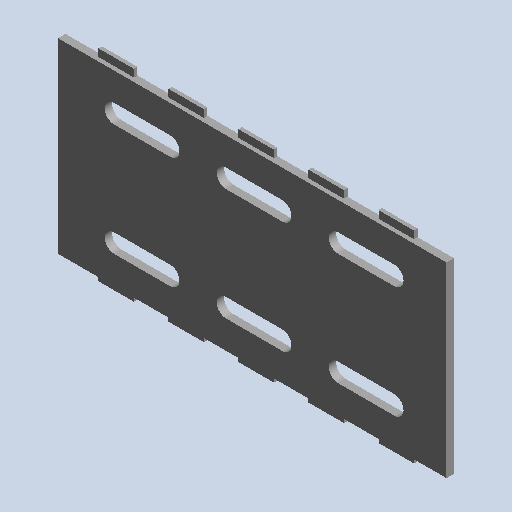
# Autodesk Inventor part: Enclosure_2
Saved by Autodesk Inventor 2026 (Build 300175050, 175E)
## iProperties
Part Number: Enclosure_2
Material: Generic
Document SubType Name: Modeling
Designer: Kartik
Mass: 75.559 g
Surface Area: 433.875 cm^2
Volume: 75.559 cm^3
Density: 1 g/cm^3
Appearance: Default
Author: Kartik
Autodesk Inventor part; units mm, degrees
ref_plane "YZ Plane" through (0, 0, 0) normal (1, 0, 0) x (0, 1, 0)
ref_plane "XZ Plane" through (0, 0, 0) normal (0, 1, 0) x (-1, 0, 0)
ref_plane "XY Plane" through (0, 0, 0) normal (0, 0, 1) x (1, 0, 0)
sketch "Sketch1" plane through (0, 0, 0) normal (0, 0, 1) x (1, 0, 0)
  line L0 (-100.0716, 53.5507) -> (107.9284, 53.5507)
  line L1 (107.9284, 53.5507) -> (107.9284, -46.4493)
  line L2 (107.9284, -46.4493) -> (-100.0716, -46.4493)
  line L3 (-100.0716, -46.4493) -> (-100.0716, 53.5507)
  point P0 (0, 0)
  dimension "d0" = 208
  dimension "d1" = 100
  constraints: 8 end point, 2 parallel, 1 horizontal, 1 perpendicular
  measures "d0" distance of L0.start L0.end
  measures "d1" distance of L0.end L1.end
extrude "Extrusion1" add sketch "Sketch1" along normal blind 4
sketch "Sketch2" plane through (-100.0716, -46.4493, 0) normal (0, -1, 0) x (1, 0, 0)
  line L0 (0, 0) -> (208, 0) projected
  line L1 (19.5, 0) -> (38.5, 0)
  line L2 (38.5, 0) -> (38.5, 1.9)
  line L3 (38.5, 1.9) -> (19.5, 1.9)
  line L4 (19.5, 1.9) -> (19.5, 0)
  line L5 (0, 0) -> (0, 4) projected
  point P0 (100.0716, 0)
  point P1 (19.5, 0.95)
  dimension "d4" = 19
  dimension "d5" = 1.9
  dimension "d6" = 19.5
  constraints: 8 end point, 2 parallel, 1 horizontal, 1 midpoint, 1 perpendicular, 1 point on line
  measures "d4" distance of L3.end L2.end
  measures "d5" distance of L2.end L1.end
  measures "d6" distance from line of L5 point (19.5, 0.95)
extrude "Extrusion2" add sketch "Sketch2" along normal blind 4
pattern_linear "Rectangular Pattern1" count 5 spacing 37.5 along (1, 0, 0) count 2 spacing 104 along (0, 1, 0) of "Extrusion2"
sketch "Sketch3" plane through (0, 0, 4) normal (0, 0, 1) x (1, 0, 0)
  line L0 (89.7284, -20.8493) -> (97.9284, -20.8493)
  line L1 (97.9284, -20.8493) -> (97.9284, -36.4493)
  line L2 (97.9284, -36.4493) -> (89.7284, -36.4493)
  line L3 (89.7284, -36.4493) -> (89.7284, -20.8493)
  line L4 (107.9284, 53.5507) -> (-100.0716, 53.5507) projected
  line L5 (-100.0716, 53.5507) -> (-100.0716, -46.4493) projected
  line L6 (107.9284, -46.4493) -> (107.9284, 53.5507) projected
  line L7 (-100.0716, -46.4493) -> (107.9284, -46.4493) projected
  point P0 (0, 0)
  dimension "d15" = 8.2
  dimension "d16" = 15.6
  dimension "d21" = 10
  dimension "d22" = 10
  constraints: 8 end point, 2 parallel, 1 horizontal, 1 perpendicular
  measures "d15" distance of L1.end L2.end
  measures "d16" distance of L0.end L1.end
  measures "d21" distance between parallel lines of L6 L1
  measures "d22" distance between parallel lines of L7 L2
extrude "Extrusion3" [suppressed]
sketch "Sketch4" plane through (0, 0, 4) normal (0, 0, 1) x (1, 0, 0)
  line L0 (-75.0716, 38.5507) -> (-35.0716, 38.5507)
  line L1 (-35.0716, 38.5507) -> (-35.0716, 28.5507)
  line L2 (-35.0716, 28.5507) -> (-75.0716, 28.5507)
  line L3 (-75.0716, 28.5507) -> (-75.0716, 38.5507)
  line L4 (-15.0716, 38.5507) -> (24.9284, 38.5507)
  line L5 (24.9284, 38.5507) -> (24.9284, 28.5507)
  line L6 (24.9284, 28.5507) -> (-15.0716, 28.5507)
  line L7 (-15.0716, 28.5507) -> (-15.0716, 38.5507)
  line L8 (44.9284, 38.5507) -> (84.9284, 38.5507)
  line L9 (84.9284, 38.5507) -> (84.9284, 28.5507)
  line L10 (84.9284, 28.5507) -> (44.9284, 28.5507)
  line L11 (44.9284, 28.5507) -> (44.9284, 38.5507)
  line L12 (-100.0716, 53.5507) -> (-100.0716, -46.4493) projected
  line L13 (107.9284, 53.5507) -> (-100.0716, 53.5507) projected
  point P0 (0, 0)
  point P1 (-75.0716, 33.5507)
  point P2 (-15.0716, 33.5507)
  point P3 (-35.0716, 33.5507)
  point P4 (44.9284, 33.5507)
  point P5 (24.9284, 33.5507)
  dimension "d23" = 40
  dimension "d24" = 10
  dimension "d25" = 40
  dimension "d26" = 10
  dimension "d27" = 40
  dimension "d28" = 10
  dimension "d29" = 25
  dimension "d30" = 20
  dimension "d31" = 20
  dimension "d35" = 15
  constraints: 24 end point, 6 parallel, 5 midpoint, 3 horizontal, 3 perpendicular, 2 point on line
  measures "d23" distance of L1.end L2.end
  measures "d24" distance of L0.end L1.end
  measures "d25" distance of L5.end L6.end
  measures "d26" distance of L4.end L5.end
  measures "d27" distance of L9.end L10.end
  measures "d28" distance of L8.end L9.end
  measures "d29" distance from line of L12 point (-75.072, 33.551)
  measures "d30" distance of point (-15.072, 33.551) point (-35.072, 33.551)
  measures "d31" distance of point (44.928, 33.551) point (24.928, 33.551)
  measures "d35" distance between parallel lines of L13 L0
extrude "Extrusion4" cut sketch "Sketch4" against normal blind 10
fillet "Fillet1" radius 5 12 edges at (-75.0716, 38.5507, 2) (-75.0716, 28.5507, 2) (-35.0716, 28.5507, 2) (-35.0716, 38.5507, 2) (-15.0716, 38.5507, 2) (-15.0716, 28.5507, 2) (24.9284, 38.5507, 2) (24.9284, 28.5507, 2) (44.9284, 38.5507, 2) (44.9284, 28.5507, 2) (84.9284, 38.5507, 2) (84.9284, 28.5507, 2)
pattern_linear "Rectangular Pattern2" count 2 spacing 60 along (0, -1, 0) of "Extrusion4", "Fillet1"
body "Solid1"
